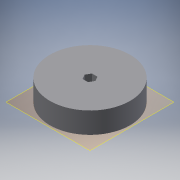
# Autodesk Inventor part: pumpSchematic
Saved by Autodesk Inventor 2017 (Build 210142000, 142)
## iProperties
Created: 2016-11-08
Part Number: pumpSchematic
Material: Generic
Document SubType Name: Modeling
Designer: Camilo
Density: 1 g/cm^3
Appearance: Default
Author: Camilo
Autodesk Inventor part; units mm, degrees
ref_plane "YZ Plane" through (0, 0, 0) normal (1, 0, 0) x (0, 1, 0)
ref_plane "XZ Plane" through (0, 0, 0) normal (0, 1, 0) x (-1, 0, 0)
ref_plane "Work Plane1" through (0, 0, 4) normal (0, 0, 1) x (1, 0, 0)
sketch "Sketch1" plane through (0, 0, 4) normal (0, 0, 1) x (1, 0, 0)
  circle A0 centre (-15.9055, -14.2497) radius 6 construction
  circle A1 centre (-15.9055, -14.2497) radius 28.486
  line L0 (-13.9713, -10.8995) -> (-12.037, -14.2497)
  line L1 (-12.037, -14.2497) -> (-13.9713, -17.6)
  line L2 (-13.9713, -17.6) -> (-17.8398, -17.6)
  line L3 (-17.8398, -17.6) -> (-19.774, -14.2497)
  line L4 (-19.774, -14.2497) -> (-17.8398, -10.8995)
  line L5 (-17.8398, -10.8995) -> (-13.9713, -10.8995)
  point P0 (0, 0)
  dimension "d0" = 56.972
  dimension "d1" = 7.737
  constraints: 12 end point, 2 centre point, 2 coincident, 1 horizontal, 13 other
  measures "d0" diameter of A1
  measures "d1" distance of L3.end L0.end
extrude "Extrusion1" add sketch "Sketch1" along normal blind 15
body "Solid1"
